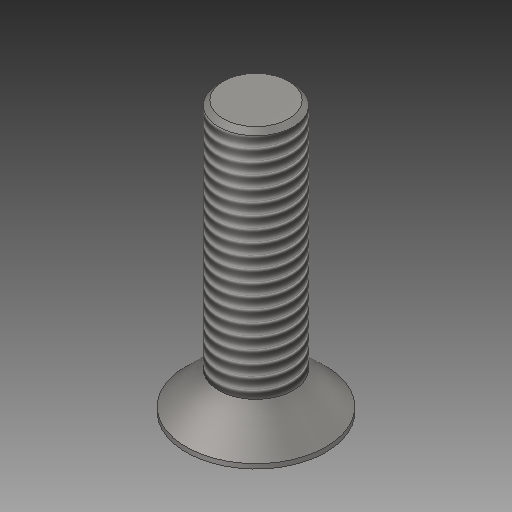
# Autodesk Inventor part: Винт М8х25 с потайной головкой
Saved by Autodesk Inventor 2019 (Build 230136000, 136)
## iProperties
Created: 2019-08-04
Part Number: Винт М8х25 с потайной головкой
Material: Сталь
Document SubType Name: Modeling
Designer: Петров Иван
Density: 7.85 g/cm^3
Appearance: Нержавеющая — шлифованная
Mass: 12.77 g
Surface Area: 11.5 cm^2
Volume: 1.62675 cm^3
Author: Петров Иван
Autodesk Inventor part; units mm, degrees
ref_plane "YZ Plane" through (0, 0, 0) normal (1, 0, 0) x (0, 1, 0)
ref_plane "XZ Plane" through (0, 0, 0) normal (0, 1, 0) x (-1, 0, 0)
ref_plane "XY Plane" through (0, 0, 0) normal (0, 0, 1) x (1, 0, 0)
sketch "Эскиз1" plane through (0, 0, 0) normal (0, 1, 0) x (-1, 0, 0)
  circle A0 centre (0, 0) radius 7.5
  dimension "d0" = 15
  constraints: 1 centre point, 1 coincident
  measures "d0" diameter of A0
extrude "Выдавливание1" add sketch "Эскиз1" along normal blind 4
sketch "Эскиз2" plane through (0, 4, 0) normal (0, 1, 0) x (1, 0, 0)
  circle A0 centre (0, 0) radius 4
  dimension "d3" = 8
  constraints: 1 centre point, 1 coincident
  measures "d3" diameter of A0
extrude "Выдавливание2" add sketch "Эскиз2" along normal blind 25
chamfer "Фаска1" distance 3.5 angle 45 1 edges at (7.5, 4, 0)
thread "Резьба1" size "M8x1.25" class "6g" standard "ANSI Metric M Profile" full length
chamfer "Фаска2" distance 0.5 angle 45 1 edges at (-4, 29, 0)
sketch "Эскиз3" plane through (0, 0, 0) normal (0, -1, 0) x (1, 0, 0)
  line L0 (-5, -1) -> (5, -1)
  line L1 (5, -1) -> (5, 1)
  line L2 (5, 1) -> (-5, 1)
  line L3 (-5, 1) -> (-5, -1)
  line L4 (-5, -1) -> (5, 1) construction
  line L5 (5, -1) -> (-5, 1) construction
  line L6 (-1, -5) -> (1, -5)
  line L7 (1, -5) -> (1, 5)
  line L8 (1, 5) -> (-1, 5)
  line L9 (-1, 5) -> (-1, -5)
  line L10 (-1, -5) -> (1, 5) construction
  line L11 (1, -5) -> (-1, 5) construction
  point P0 (0, 0)
  dimension "d14" = 10
  dimension "d15" = 2
  dimension "d16" = 10
  dimension "d17" = 2
  constraints: 24 end point, 4 midpoint, 4 parallel, 2 horizontal, 2 perpendicular
  measures "d14" distance of L2.end L1.end
  measures "d15" distance of L8.end L7.end
  measures "d16" distance of L6.end L7.end
  measures "d17" distance of L0.end L1.end
extrude "Выдавливание3" cut sketch "Эскиз3" against normal blind 2.5
